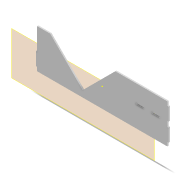
# Autodesk Inventor part: Frontal
Saved by Autodesk Inventor 2022 (Build 260153000, 153)
## iProperties
Created: 2022-06-06
Part Number: Frontal
Material: Generic
Document SubType Name: Modeling
Designer: ADMIN
Density: 1 g/cm^3
Appearance: Default
Author: ADMIN
Autodesk Inventor part; units mm, degrees
ref_plane "YZ Plane" through (0, 0, 0) normal (1, 0, 0) x (0, 1, 0)
ref_plane "XZ Plane" through (0, 0, 0) normal (0, 1, 0) x (-1, 0, 0)
ref_plane "XY Plane" through (0, 0, 0) normal (0, 0, 1) x (1, 0, 0)
ref_plane "Work Plane1" through (-2219.9027, -150.7269, 0) normal (0, 0, 1) x (1, 0, 0)
sketch "Sketch1" plane through (-2219.9027, -150.7269, 0) normal (0, 0, 1) x (1, 0, 0)
  line L0 (1984.9027, 130.3224) -> (1984.9027, 75.7269) projected
  line L1 (1984.9027, 75.7269) -> (2354.9027, 75.7269) projected
  line L2 (2354.9027, 75.7269) -> (2354.9027, 130.3224) projected
  line L3 (2354.9027, 130.3224) -> (2369.9027, 130.3224) projected
  line L4 (2369.9027, 130.3224) -> (2369.9027, 225.7269) projected
  line L5 (2369.9027, 225.7269) -> (2354.9027, 225.7269) projected
  line L6 (1969.9027, 225.7269) -> (1969.9027, 130.3224) projected
  line L7 (1969.9027, 130.3224) -> (1984.9027, 130.3224) projected
  line L8 (1969.9027, 160.7269) -> (1969.9027, 210.7269) projected
  line L9 (1969.9027, 210.7269) -> (1964.9027, 210.7269) projected
  line L10 (1964.9027, 160.7269) -> (1964.9027, 210.7269) projected
  line L11 (1969.9027, 160.7269) -> (1964.9027, 160.7269) projected
  line L12 (1969.9027, 90.7269) -> (1969.9027, 140.7269) projected
  line L13 (1969.9027, 140.7269) -> (1964.9027, 140.7269) projected
  line L14 (1964.9027, 90.7269) -> (1964.9027, 140.7269) projected
  line L15 (1969.9027, 90.7269) -> (1964.9027, 90.7269) projected
  line L16 (1964.9027, 160.7269) -> (1969.9027, 160.7269)
  line L17 (1969.9027, 160.7269) -> (1969.9027, 140.7269)
  line L18 (1969.9027, 140.7269) -> (1964.9027, 140.7269)
  line L19 (1964.9027, 140.7269) -> (1964.9027, 160.7269)
  line L20 (1991.136, 206.6179) -> (1964.9027, 206.6179)
  line L21 (1964.9027, 206.6179) -> (1964.9027, 210.7269)
  line L22 (1964.9027, 210.7269) -> (1991.136, 210.7269)
  line L23 (1991.136, 210.7269) -> (1991.136, 206.6179)
  line L24 (1964.9027, 90.7269) -> (1991.136, 90.7269)
  line L25 (1991.136, 90.7269) -> (1991.136, 75.7269)
  line L26 (1991.136, 75.7269) -> (1964.9027, 75.7269)
  line L27 (1964.9027, 75.7269) -> (1964.9027, 90.7269)
  line L28 (1984.9027, 75.7269) -> (1969.9027, 75.7269)
  line L29 (1969.9027, 75.7269) -> (1969.9027, 130.3224)
  line L30 (1969.9027, 130.3224) -> (1984.9027, 130.3224)
  line L31 (1984.9027, 130.3224) -> (1984.9027, 75.7269)
  line L32 (2374.9027, 160.7269) -> (2374.9027, 210.7269) projected
  line L33 (2374.9027, 210.7269) -> (2369.9027, 210.7269) projected
  line L34 (2369.9027, 160.7269) -> (2369.9027, 210.7269) projected
  line L35 (2374.9027, 160.7269) -> (2369.9027, 160.7269) projected
  line L36 (2374.9027, 90.7269) -> (2374.9027, 140.7269) projected
  line L37 (2374.9027, 140.7269) -> (2369.9027, 140.7269) projected
  line L38 (2369.9027, 90.7269) -> (2369.9027, 140.7269) projected
  line L39 (2374.9027, 90.7269) -> (2369.9027, 90.7269) projected
  line L40 (2369.9027, 75.7269) -> (2354.9027, 75.7269)
  line L41 (2354.9027, 75.7269) -> (2354.9027, 130.3224)
  line L42 (2354.9027, 130.3224) -> (2369.9027, 130.3224)
  line L43 (2369.9027, 130.3224) -> (2369.9027, 75.7269)
  line L44 (2269.9027, 225.7269) -> (2243.8976, 199.7218) projected
  line L45 (2144.9027, 100.7269) -> (2109.5473, 136.0822) projected
  line L46 (2019.9027, 225.7269) -> (2007.4027, 225.7269) projected
  line L47 (2183.7935, 132.5467) -> (2180.258, 136.0822) projected
  line L48 (2180.258, 136.0822) -> (2144.9027, 100.7269) projected
  line L49 (2109.5473, 136.0822) -> (2106.0118, 132.5467) projected
  line L50 (2106.0118, 132.5467) -> (2084.7986, 153.7599) projected
  line L51 (2084.7986, 153.7599) -> (2088.3341, 157.2954) projected
  line L52 (2088.3341, 157.2954) -> (2067.1209, 178.5086) projected
  line L53 (2067.1209, 178.5086) -> (2063.5854, 174.9731) projected
  line L54 (2063.5854, 174.9731) -> (2042.3722, 196.1863) projected
  line L55 (2042.3722, 196.1863) -> (2045.9077, 199.7218) projected
  line L56 (2045.9077, 199.7218) -> (2019.9027, 225.7269) projected
  line L57 (2243.8976, 199.7218) -> (2247.4332, 196.1863) projected
  line L58 (2247.4332, 196.1863) -> (2226.22, 174.9731) projected
  line L59 (2226.22, 174.9731) -> (2222.6844, 178.5086) projected
  line L60 (2222.6844, 178.5086) -> (2201.4712, 157.2954) projected
  line L61 (2201.4712, 157.2954) -> (2205.0068, 153.7599) projected
  line L62 (2205.0068, 153.7599) -> (2183.7935, 132.5467) projected
  line L63 (2329.9027, 220.7269) -> (2329.9027, 225.7269) projected
  line L64 (2329.9027, 225.7269) -> (2309.9027, 225.7269) projected
  line L65 (2309.9027, 225.7269) -> (2309.9027, 220.7269) projected
  line L66 (2309.9027, 220.7269) -> (2284.9027, 220.7269) projected
  line L67 (2284.9027, 220.7269) -> (2284.9027, 225.7269) projected
  line L68 (2284.9027, 225.7269) -> (2269.9027, 225.7269) projected
  line L69 (2007.4027, 225.7269) -> (2007.4027, 220.7269) projected
  line L70 (2007.4027, 220.7269) -> (1982.4027, 220.7269) projected
  line L71 (1982.4027, 220.7269) -> (1982.4027, 225.7269) projected
  line L72 (1982.4027, 225.7269) -> (1969.9027, 225.7269) projected
  line L73 (2354.9027, 225.7269) -> (2354.9027, 220.7269) projected
  line L74 (2354.9027, 220.7269) -> (2329.9027, 220.7269) projected
  point P0 (2219.9027, 150.7269)
  point P1 (1991.136, 21.6179)
  point P2 (1991.136, 6.6179)
  point P3 (1969.9027, 90.7269)
  point P4 (820.3787, 21.6179)
  point P5 (1320.3787, 21.6179)
  point P6 (820.3787, 20.4045)
  point P7 (1984.9027, 75.7269)
  point P8 (1305.3787, -34.1911)
  point P9 (820.3787, 21.6179)
  point P10 (2369.9027, 90.7269)
  point P11 (2369.9027, 130.3224)
  point P12 (2354.9027, 75.7269)
  point P13 (1969.9027, 206.6179)
  constraints: 40 end point, 10 parallel, 5 horizontal, 5 perpendicular, 1 collinear, 1 point on line
extrude "Extrusion1" add sketch "Sketch1" along normal blind 5 contours L7 L6 L20 L23 L22 L72 L71 L70 L69 L46 L56 L55 L54 L53 L52 L51 L50 L49 L45 L48 L47 L62 L61 L60 L59 L58 L57 L44 L68 L67 L66 L65 L64 L63 L74 L73 L5 L4 L3 L2 L1 L25 L24 L0 | L0 L24 L12 L7 | L24 L25 L1 L0 | L0 L26 L29 L24 | L12 L15 L14 L13 L6 | L11 L10 L20 L6 | L2 L3 L38 L43 L40 | L6 L22 L23 L20 | L4 L37 L36 L39 L38 | L4 L33 L32 L35
sketch "Sketch3" plane through (-2219.9027, -150.7269, 5) normal (0, 0, 1) x (1, 0, 0)
  point P0 (2219.9027, 150.7269)
sketch "Sketch4" plane through (-2219.9027, -150.7269, 5) normal (0, 0, 1) x (1, 0, 0)
  line L0 (2284.9027, 160.7269) -> (2309.9027, 160.7269)
  line L1 (2309.9027, 160.7269) -> (2309.9027, 155.7269)
  line L2 (2309.9027, 155.7269) -> (2284.9027, 155.7269)
  line L3 (2284.9027, 155.7269) -> (2284.9027, 160.7269)
  line L4 (1969.9027, 225.7269) -> (1969.9027, 206.6179) projected
  line L5 (1969.9027, 160.7269) -> (1969.9027, 140.7269) projected
  line L6 (1969.9027, 140.7269) -> (1964.9027, 140.7269) projected
  line L7 (1964.9027, 140.7269) -> (1964.9027, 90.7269) projected
  line L8 (1969.9027, 75.7269) -> (2369.9027, 75.7269) projected
  line L9 (2369.9027, 90.7269) -> (2374.9027, 90.7269) projected
  line L10 (2374.9027, 90.7269) -> (2374.9027, 140.7269) projected
  line L11 (2374.9027, 140.7269) -> (2369.9027, 140.7269) projected
  line L12 (2369.9027, 140.7269) -> (2369.9027, 160.7269) projected
  line L13 (2369.9027, 160.7269) -> (2374.9027, 160.7269) projected
  line L14 (2374.9027, 160.7269) -> (2374.9027, 210.7269) projected
  line L15 (2374.9027, 210.7269) -> (2369.9027, 210.7269) projected
  line L16 (2369.9027, 210.7269) -> (2369.9027, 225.7269) projected
  line L17 (2369.9027, 225.7269) -> (2354.9027, 225.7269) projected
  line L18 (2329.9027, 160.7269) -> (2354.9027, 160.7269)
  line L19 (2354.9027, 160.7269) -> (2354.9027, 155.7269)
  line L20 (2354.9027, 155.7269) -> (2329.9027, 155.7269)
  line L21 (2329.9027, 155.7269) -> (2329.9027, 160.7269)
  line L22 (2269.9027, 225.7269) -> (2243.8976, 199.7218) projected
  line L23 (2144.9027, 100.7269) -> (2109.5473, 136.0822) projected
  line L24 (2019.9027, 225.7269) -> (2007.4027, 225.7269) projected
  line L25 (1964.9027, 90.7269) -> (1969.9027, 90.7269) projected
  line L26 (2369.9027, 75.7269) -> (2369.9027, 90.7269) projected
  line L27 (1969.9027, 90.7269) -> (1969.9027, 75.7269) projected
  line L28 (1969.9027, 206.6179) -> (1964.9027, 206.6179) projected
  line L29 (1964.9027, 206.6179) -> (1964.9027, 160.7269) projected
  line L30 (1964.9027, 160.7269) -> (1969.9027, 160.7269) projected
  line L31 (2243.8976, 199.7218) -> (2247.4332, 196.1863) projected
  line L32 (2247.4332, 196.1863) -> (2226.22, 174.9731) projected
  line L33 (2226.22, 174.9731) -> (2222.6844, 178.5086) projected
  line L34 (2222.6844, 178.5086) -> (2201.4712, 157.2954) projected
  line L35 (2201.4712, 157.2954) -> (2205.0068, 153.7599) projected
  line L36 (2205.0068, 153.7599) -> (2183.7935, 132.5467) projected
  line L37 (2183.7935, 132.5467) -> (2180.258, 136.0822) projected
  line L38 (2180.258, 136.0822) -> (2144.9027, 100.7269) projected
  line L39 (2109.5473, 136.0822) -> (2106.0118, 132.5467) projected
  line L40 (2106.0118, 132.5467) -> (2084.7986, 153.7599) projected
  line L41 (2084.7986, 153.7599) -> (2088.3341, 157.2954) projected
  line L42 (2088.3341, 157.2954) -> (2067.1209, 178.5086) projected
  line L43 (2067.1209, 178.5086) -> (2063.5854, 174.9731) projected
  line L44 (2063.5854, 174.9731) -> (2042.3722, 196.1863) projected
  line L45 (2042.3722, 196.1863) -> (2045.9077, 199.7218) projected
  line L46 (2045.9077, 199.7218) -> (2019.9027, 225.7269) projected
  line L47 (2354.9027, 225.7269) -> (2354.9027, 220.7269) projected
  line L48 (2354.9027, 220.7269) -> (2329.9027, 220.7269) projected
  line L49 (2329.9027, 220.7269) -> (2329.9027, 225.7269) projected
  line L50 (2329.9027, 225.7269) -> (2309.9027, 225.7269) projected
  line L51 (2309.9027, 225.7269) -> (2309.9027, 220.7269) projected
  line L52 (2309.9027, 220.7269) -> (2284.9027, 220.7269) projected
  line L53 (2284.9027, 220.7269) -> (2284.9027, 225.7269) projected
  line L54 (2284.9027, 225.7269) -> (2269.9027, 225.7269) projected
  line L55 (2007.4027, 225.7269) -> (2007.4027, 220.7269) projected
  line L56 (2007.4027, 220.7269) -> (1982.4027, 220.7269) projected
  line L57 (1982.4027, 220.7269) -> (1982.4027, 225.7269) projected
  line L58 (1982.4027, 225.7269) -> (1969.9027, 225.7269) projected
  point P0 (2219.9027, 150.7269)
  dimension "d16" = 25
  dimension "d17" = 5
  dimension "d18" = 80
  dimension "d19" = 25
  dimension "d20" = 5
  dimension "d22" = 15
  dimension "d25" = 20
  constraints: 16 end point, 4 parallel, 2 horizontal, 2 perpendicular, 1 collinear
  measures "d16" distance of L1.end L2.end
  measures "d17" distance of L0.end L1.end
  measures "d18" distance between parallel lines of L8 L2
  measures "d19" distance of L19.end L20.end
  measures "d20" distance of L18.end L19.end
  measures "d22" distance between parallel lines of L12 L19
  measures "d25" distance between parallel lines of L21 L1
extrude "Extrusion3" cut sketch "Sketch4" against normal blind 5 contours L0 L1 L2 L3 | L18 L19 L20 L21
equation "\"d19\" = d16"
body "Solid1"
